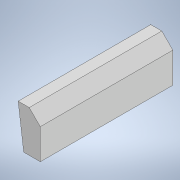
# Autodesk Inventor part: outside-join-half-old
Saved by Autodesk Inventor 2021 (Build 250183000, 183)
## iProperties
Created: 2020-12-10
Part Number: outside-join-half-old
Material: Generic
Document SubType Name: Modeling
Designer: Luke Kamols
Density: 1 g/cm^3
Appearance: Default
Author: Luke Kamols
Autodesk Inventor part; units mm, degrees
ref_plane "YZ Plane" through (0, 0, 0) normal (1, 0, 0) x (0, 1, 0)
ref_plane "XZ Plane" through (0, 0, 0) normal (0, 1, 0) x (-1, 0, 0)
ref_plane "XY Plane" through (0, 0, 0) normal (0, 0, 1) x (1, 0, 0)
sketch "Sketch1" plane through (0, 0, 0) normal (0, 0, 1) x (1, 0, 0)
  line L0 (0, 0) -> (6, 0)
  line L1 (6, 0) -> (6, 11)
  line L2 (0, 15) -> (2, 15)
  line L3 (2, 15) -> (6, 11)
  line L4 (0, 15) -> (-2, 15)
  line L5 (-2, 15) -> (0, 0)
  dimension "d0" = 6
  dimension "d1" = 11
  dimension "d2" = 15
  dimension "d4" = 2
  dimension "d5" = 2
  constraints: 12 end point, 3 horizontal, 1 perpendicular
  measures "d0" distance of L0.start L0.end
  measures "d1" distance of L0.end L1.end
  measures "d2" distance of L0.start L2.start
  measures "d4" distance of L2.start L2.end
  measures "d5" distance of L2.start L4.end
extrude "Extrusion1" add sketch "Sketch1" along normal blind 10
sketch "Sketch2" plane through (0, 0, 10) normal (0, 0, 1) x (1, 0, 0)
  line L0 (6, 0) -> (6, 11) projected
  line L1 (6, 0) -> (6, 11)
  line L2 (6, 11) -> (2, 15) projected
  line L3 (6, 11) -> (2, 15)
  line L4 (-2, 15) -> (0, 0) projected
  line L5 (2, 15) -> (-2, 15)
  line L6 (0, 0) -> (6, 0) projected
  line L7 (6, 0) -> (3, 0)
  line L8 (0, 11) -> (3, 0)
  line L9 (-3, 0) -> (0, 11)
  line L10 (-6, 11) -> (-2, 15)
  line L11 (-5, 0) -> (-6, 4)
  line L12 (-3, 0) -> (-5, 0)
  line L13 (-6, 4) -> (-6, 11)
  point P0 (-0.9851, 7.3881)
  dimension "d9" = 3
  constraints: 20 end point, 2 collinear, 2 horizontal, 1 midpoint, 1 vertical
  measures "d9" distance of L4.end L9.start
extrude "Extrusion2" add sketch "Sketch2" along normal blind 28 contours L6 L8 L9 L4 L5 L2 L0 | L4 L9 L12 L11 L13 L10
sketch "Sketch3" plane through (0, 0, 38) normal (0, 0, 1) x (1, 0, 0)
  line L0 (-2, 15) -> (0, 0) projected
  line L1 (2, 15) -> (-2, 15) projected
  line L2 (6, 11) -> (2, 15) projected
  line L3 (6, 0) -> (6, 11) projected
  line L4 (0, 0) -> (6, 0) projected
extrude "Extrusion3" add sketch "Sketch3" along normal blind 10
sketch "Sketch6" plane through (6, 0, 0) normal (1, 0, 0) x (0, 0, -1)
  line L0 (0, 15) -> (0, 0) projected
  line L1 (0, 0) -> (-10, 0) projected
  line L2 (0, 0) -> (-10, 0)
  line L3 (-10, 15) -> (-10, 7.3881) projected
  line L4 (-10, 0) -> (-10, 15)
  line L5 (-10, 15) -> (-8, 15)
  line L6 (0, 15) -> (-10, 15) projected
  line L7 (-10, 7.3881) -> (-10, 0) projected
  line L8 (-8, 15) -> (-10, 0)
  line L9 (-10, 0) -> (-10.3965, 0.0529)
  dimension "d19" = 15
  dimension "d20" = 2
  dimension "d36" = 0.4
  constraints: 10 end point, 2 perpendicular, 1 collinear, 1 point on line
  measures "d19" distance of L1.end L3.start
  measures "d20" distance of L3.start L5.end
  measures "d36" distance of L1.end L9.end
extrude "Extrusion4" cut sketch "Sketch6" against normal blind 33.8125 contours L8 L4 L3 L5
sketch "Sketch7" plane through (0, 0, 10) normal (0, 0, -1) x (-1, 0, 0)
  line L0 (3, 0) -> (0, 11) projected
  line L1 (5, 0) -> (3, 0) projected
  line L2 (6, 4) -> (5, 0) projected
  line L3 (6, 11) -> (6, 4) projected
  line L4 (2, 15) -> (6, 11) projected
  line L5 (-2, 15) -> (2, 15) projected
  line L6 (-6, 11) -> (-2, 15) projected
  line L7 (-6, 0) -> (-6, 11) projected
  line L8 (-3, 0) -> (-6, 0) projected
  line L9 (-3, 0) -> (0, 11) projected
  point P0 (0, 0)
extrude "Extrusion5" add sketch "Sketch7" along normal up to surface surface through (6, 15, 8) normal (0, -0.1321637, -0.9912279)
sketch "Sketch8" plane through (0, 0, 38) normal (0, 0, -1) x (-1, 0, 0)
  line L0 (0, 11) -> (-3, 0) projected
  line L1 (0, 0) -> (-3, 0) projected
  line L2 (0.9851, 7.3881) -> (0, 0) projected
  line L3 (0.9851, 7.3881) -> (0, 11) projected
extrude "Extrusion6" cut sketch "Sketch8" along normal blind 30 and the other way blind 2
sketch "Sketch10" plane through (6, 0, 0) normal (1, 0, 0) x (0, 0, -1)
  line L0 (-48, 15) -> (-48, 0) projected
  line L1 (-48, 0) -> (-38, 0)
  line L2 (0, 0) -> (-48, 0) projected
  line L3 (-38, 7.3881) -> (-38, 15) projected
  line L4 (-38, 0) -> (-38, 15)
  line L5 (-8, 15) -> (-38, 15) projected
  line L6 (-38, 15) -> (-40, 15)
  line L7 (0, 15) -> (-48, 15) projected
  line L8 (-40, 15) -> (-38, 0)
  dimension "d29" = 10
  dimension "d33" = 2
  constraints: 8 end point, 2 point on line
  measures "d29" distance of L0.end L1.end
  measures "d33" distance of L3.end L6.end
extrude "Extrusion7" cut sketch "Sketch10" against normal blind 17.625 contours L6 L3 L4 L8
sketch "Sketch12" plane through (0, 0, 38) normal (0, 0, 1) x (1, 0, 0)
  line L0 (-2, 15) -> (-6, 11) projected
  line L1 (-6, 11) -> (-6, 4) projected
  line L2 (-6, 4) -> (-5, 0) projected
  line L3 (-5, 0) -> (-3, 0) projected
  line L4 (-3, 0) -> (0, 11) projected
  line L5 (3, 0) -> (0, 11) projected
  line L6 (3, 0) -> (6, 0) projected
  line L7 (6, 11) -> (6, 0) projected
  line L8 (2, 15) -> (6, 11) projected
  line L9 (-2, 15) -> (2, 15) projected
  point P0 (0, 0)
extrude "Extrusion8" add sketch "Sketch12" along normal up to surface surface through (6, 0, 38) normal (0, -0.1321637, 0.9912279)
body "Solid1"
